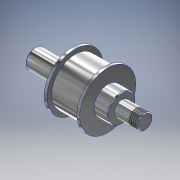
# Autodesk Inventor part: Puleggia minore
Saved by Autodesk Inventor 2018 (Build 220112000, 112)
## iProperties
Created: 2020-06-04
Part Number: Puleggia minore
Material: Alluminio 6061
Document SubType Name: Modeling
Designer: Francesco
Density: 2.7 g/cm^3
Appearance: Alluminio - Piatto
Mass: 237.466 g
Surface Area: 170.369 cm^2
Volume: 87.9503 cm^3
Author: Francesco
Autodesk Inventor part; units mm, degrees
ref_plane "YZ Plane" through (0, 0, 0) normal (1, 0, 0) x (0, 1, 0)
ref_plane "XZ Plane" through (0, 0, 0) normal (0, 1, 0) x (-1, 0, 0)
ref_plane "XY Plane" through (0, 0, 0) normal (0, 0, 1) x (1, 0, 0)
sketch "Schizzo1" plane through (0, 0, 0) normal (0, 0, 1) x (1, 0, 0)
  line L0 (-16, 25) -> (16, 25)
  line L1 (-16, 25) -> (-16, 32)
  line L2 (-16, 32) -> (-19, 32)
  line L3 (-19, 32) -> (-19, 0)
  line L4 (16, 25) -> (16, 32)
  line L5 (16, 32) -> (19, 32)
  line L6 (19, 32) -> (19, 0)
  line L7 (-19, 0) -> (19, 0)
  point P0 (0, 0)
  point P1 (0, 0)
  dimension "d2" = 7
  dimension "d3" = 3
  dimension "d4" = 3
  dimension "d5" = 7
  dimension "d6" = 50
  dimension "d7" = 32
  dimension "d8" = 38
  constraints: 16 end point, 3 perpendicular, 2 horizontal, 2 vertical, 1 coincident, 1 horizontal alignment, 1 midpoint
  measures "d2" distance of L0.start L1.end
  measures "d3" distance of L1.end L2.end
  measures "d4" distance of L4.end L5.end
  measures "d5" distance between parallel lines of L0 L5
  measures "d6" diameter of L0 L7
  measures "d7" distance between parallel lines of L4 L1
  measures "d8" distance between parallel lines of L6 L3
revolve "Rivoluzione1" add sketch "Schizzo1" angle 360 about axis through (-19, 0, 0) along (1, 0, 0)
sketch "Schizzo3" plane through (-19, 0, 0) normal (-1, 0, 0) x (0, 0, 1)
  point P0 (0, 0)
sketch "Schizzo4" plane through (19, 0, 0) normal (1, 0, 0) x (0, 0, -1)
  circle A0 centre (0, 0) radius 14.75
  dimension "d13" = 29.5
  constraints: 1 centre point, 1 coincident
  measures "d13" diameter of A0
extrude "Estrusione2" add sketch "Schizzo4" along normal blind 15
sketch "Schizzo5" plane through (34, 0, 0) normal (1, 0, 0) x (0, 0, -1)
  circle A0 centre (0, 0) radius 8
  dimension "d16" = 16
  constraints: 1 centre point, 1 coincident
  measures "d16" diameter of A0
extrude "Estrusione3" add sketch "Schizzo5" along normal blind 25
thread "Filettatura1" size "M16x2" class "6g" standard "ANSI Metric M Profile" length 10
sketch "Schizzo6" plane through (-19, 0, 0) normal (-1, 0, 0) x (0, 0, 1)
  circle A0 centre (0, 0) radius 10
  dimension "d24" = 20
  constraints: 1 centre point, 1 coincident
  measures "d24" diameter of A0
extrude "Estrusione4" add sketch "Schizzo6" along normal blind 40
chamfer "Smusso1" distance 0.75 angle 45 3 edges at (34, 0, 14.75) (59, 0, 8) (-59, 0, -10)
